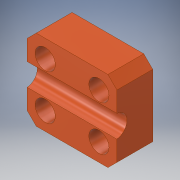
# Autodesk Inventor part: Driver Clamp 2
Saved by Autodesk Inventor 2018 (Build 220112000, 112)
## iProperties
Created: 2013-11-24
Part Number: Driver Clamp 2
Material: ABS Plastic
Document SubType Name: Modeling
Designer: Gabriel Smolnycki
Mass: 2.26381 g
Surface Area: 16.3009 cm^2
Volume: 2.13567 cm^3
Density: 1.06 g/cm^3
Appearance: Smooth - Light Orange
Author: Gabriel Smolnycki
Sending System: SolidWorks 2017
Last Author: Gabriel Smolnycki
Last Saved: 2017-09-14
Autodesk Inventor part; units mm, degrees
ref_plane "YZ Plane" through (0, 0, 0) normal (1, 0, 0) x (0, 1, 0)
ref_plane "XZ Plane" through (0, 0, 0) normal (0, 1, 0) x (-1, 0, 0)
sketch "Sketch1" plane through (0, 0, 0) normal (0, 0, 1) x (1, 0, 0)
  line L0 (8, -9) -> (10, -7)
  line L1 (10, -7) -> (10, 7)
  line L2 (-10, 7) -> (-10, -7)
  line L3 (10, 7) -> (8, 9)
  line L4 (-10, -7) -> (-8, -9)
  line L5 (8, 9) -> (-8, 9)
  line L6 (-8, -9) -> (8, -9)
  line L7 (-8, 9) -> (-10, 7)
  constraints: 16 end point, 5 equal length, 2 horizontal, 2 vertical, 1 perpendicular
extrude "Extrusion1" add sketch "Sketch1" along normal blind 8
ref_plane "Work Plane1" through (-10.001, 0, 8.25) normal (0, 0.1, 0.995) x (1, 0, 0)
sketch "Sketch2" plane through (-10.001, 0, 8.25) normal (0, 0.1, 0.995) x (1, 0, 0)
  line L0 (20.001, 2.5) -> (0.001, 2.5)
  line L1 (20.001, 2.5) -> (20.001, 0)
  line L2 (0.001, 2.5) -> (0.001, 0)
  line L3 (20.001, 0) -> (0.001, 0)
  line L4 (0, 0) -> (10, 0)
  constraints: 10 end point, 3 horizontal, 2 vertical, 1 collinear
revolve "Revolution1" cut sketch "Sketch2" angle 168.522 about axis through (-10.001, 0, 8.25) along (-1, 0, 0)
hole "Hole4" at (6, -5, 8) direction (0, 0, -1) diameter 4.5 depth 8
hole "Hole3" at (-6, -5, 8) direction (0, 0, -1) diameter 4.5 depth 8
sketch "Sketch4" plane through (0, 0, 8) normal (0, 0, 1) x (1, 0, 0)
  point P0 (-6, -5)
hole "Hole2" at (6, 5, 8) direction (0, 0, -1) diameter 4.5 depth 8
sketch "Sketch3" plane through (0, 0, 8) normal (0, 0, 1) x (1, 0, 0)
  point P0 (6, -5)
hole "Hole1" at (-6, 5, 8) direction (0, 0, -1) diameter 4.5 depth 8
sketch "Sketch5" plane through (0, 0, 8) normal (0, 0, 1) x (1, 0, 0)
  point P0 (6, 5)
sketch "Sketch6" plane through (0, 0, 8) normal (0, 0, 1) x (1, 0, 0)
  point P0 (-6, 5)
body "Solid3"
